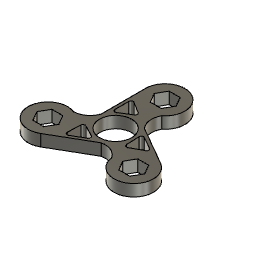
fidget-spinner (Autodesk Fusion 360 design; units mm, degrees)
Autodesk Fusion 360 part; units mm, degrees
note: some values were not read from the file. Set by a fixed rule: which sketch regions a step uses.
sketch "Sketch1" plane through (0, 0, 0) normal (0, 0, 1) x (1, 0, 0)
  circle A0 centre (0, 0) radius 4
  circle A1 centre (0, 0) radius 11
  line L0 (3.7528, 27.5) -> (7.5056, 34)
  line L1 (7.5056, 34) -> (3.7528, 40.5)
  line L2 (3.7528, 40.5) -> (-3.7528, 40.5)
  line L3 (-3.7528, 40.5) -> (-7.5056, 34)
  line L4 (-7.5056, 34) -> (-3.7528, 27.5)
  line L5 (-3.7528, 27.5) -> (3.7528, 27.5)
  line L6 (0, 0) -> (0, -80) construction
  circle A2 centre (0, 0) radius 48 construction
  circle A3 centre (0, 34) radius 13.5
  line L7 (-13.5, 34) -> (-13.5, 3.6173)
  arc A4 (8.2813, 23.3384) -> (9.8827, 9.8827) centre (18.6421, 17.7483) ccw
  line L8 (-22.6949, -28.6913) -> (3.6173, -13.5)
  circle A5 centre (-29.4449, -17) radius 13.5
  line L9 (-36.9504, -17) -> (-33.1976, -23.5)
  line L10 (-33.1976, -23.5) -> (-25.6921, -23.5)
  line L11 (-25.6921, -23.5) -> (-21.9393, -17)
  line L12 (-21.9393, -17) -> (-25.6921, -10.5)
  line L13 (-33.1976, -10.5) -> (-36.9504, -17)
  line L14 (-25.6921, -10.5) -> (-33.1976, -10.5)
  arc A6 (-24.3523, -4.4974) -> (-13.5, 3.6173) centre (-24.6915, 7.2704) ccw
  line L15 (36.1949, -5.3087) -> (9.8827, 9.8827)
  circle A7 centre (29.4449, -17) radius 13.5
  line L16 (33.1976, -23.5) -> (36.9504, -17)
  line L17 (36.9504, -17) -> (33.1976, -10.5)
  line L18 (33.1976, -10.5) -> (25.6921, -10.5)
  line L19 (25.6921, -10.5) -> (21.9393, -17)
  line L20 (25.6921, -23.5) -> (33.1976, -23.5)
  line L21 (21.9393, -17) -> (25.6921, -23.5)
  arc A8 (16.071, -18.841) -> (3.6173, -13.5) centre (6.0494, -25.0187) ccw
  line L22 (0, 11) -> (0, 20.5)
  line L23 (-11.5, 15.75) -> (-11.5, 20.5436)
  line L24 (-11.5, 15.75) -> (-11.5, 10.9564)
  line L25 (-9.205, 21.8156) -> (-1.5352, 17.022)
  line L26 (-1.5352, 14.478) -> (-9.205, 9.6844)
  arc A9 (-9.205, 21.8156) -> (-11.5, 20.5436) centre (-10, 20.5436) ccw
  arc A10 (-1.5352, 14.478) -> (-1.5352, 17.022) centre (-2.3302, 15.75) ccw
  arc A11 (-11.5, 10.9564) -> (-9.205, 9.6844) centre (-10, 10.9564) ccw
  arc A12 (-3.7385, -15.4375) -> (-3.7844, -12.814) centre (-4.4885, -14.1384) ccw
  line L27 (-7.8899, -17.8343) -> (-3.7385, -15.4375)
  line L28 (-7.8899, -17.8343) -> (-12.0413, -20.2311)
  arc A13 (-14.2904, -18.8796) -> (-12.0413, -20.2311) centre (-12.7913, -18.9321) ccw
  line L29 (-14.2904, -18.8796) -> (-13.9739, -9.8405)
  arc A14 (-11.7707, -8.5685) -> (-13.9739, -9.8405) centre (-12.4748, -9.893) ccw
  line L30 (-11.7707, -8.5685) -> (-3.7844, -12.814)
  arc A15 (15.2385, 4.4811) -> (12.9894, 3.1296) centre (14.4885, 3.1821) ccw
  line L31 (19.3899, 2.0843) -> (15.2385, 4.4811)
  line L32 (19.3899, 2.0843) -> (23.5413, -0.3125)
  arc A16 (23.4954, -2.936) -> (23.5413, -0.3125) centre (22.7913, -1.6116) ccw
  line L33 (23.4954, -2.936) -> (15.5091, -7.1815)
  arc A17 (13.3059, -5.9095) -> (15.5091, -7.1815) centre (14.805, -5.857) ccw
  line L34 (13.3059, -5.9095) -> (12.9894, 3.1296)
  point P0 (0, 36)
  point P1 (-11.5, 23.25)
  point P2 (-11.5, 8.25)
  point P3 (0.5, 15.75)
  dimension "d25" = 13.5
  dimension "d46" = 22
  dimension "d47" = 96
  dimension "d51" = 12
  dimension "d52" = 1.5
  dimension "d53" = 1.5
  dimension "d54" = 1.5
  dimension "d56" = 360
  constraint coincident A0.centre A1.centre
  constraint horizontal L2
  constraint vertical L6
  constraint concentric A1 A2
  constraint coincident A3 L7.start
  constraint tangent A3 L7
  constraint coincident A3 A4.start
  constraint coincident A7 A8.start
  constraint coincident A5 A6.start
  constraint coincident A1 L22.start
  constraint coincident A3 L22.end
  constraint vertical L22
  constraint coincident P1 L23
  constraint coincident P1 L25
  constraint tangent L23 A9
  constraint tangent L25 A9
  constraint coincident P3 L25
  constraint coincident P3 L26
  constraint tangent L25 A10
  constraint tangent L26 A10
  constraint coincident P2 L24
  constraint coincident P2 L26
  constraint tangent L24 A11
  constraint tangent L26 A11
  measures "d25" radius of A3
  measures "d46" diameter of A1
  measures "d47" diameter of A2
  measures "d51" distance of L23.start P3
  measures "d52" radius of A9
  measures "d53" radius of A10
  measures "d54" radius of A11
extrude "Extrude1" add sketch "Sketch1" along normal blind 8 contours A3 | A3 L7 A4 L8 A5 A6 L15 A7 A8 | A5 | A7 makes body 1
copy_body "Body->Comp1" bodies 1 removing the originals makes body 2 in component "Component"
component "Component" placed x (1, 0, 0) y (0, 1, 0) z (0, 0, 1) at (0, 0, 0)
